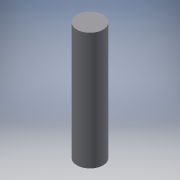
# Autodesk Inventor part: cil_sierra
Saved by Autodesk Inventor 2018 (Build 220112000, 112)
## iProperties
Created: 2021-07-10
Part Number: cil_sierra
Material: Genérico
Document SubType Name: Modeling
Designer: GABRIEL
Density: 1 g/cm^3
Appearance: Valor por defecto
Author: GABRIEL
Autodesk Inventor part; units mm, degrees
ref_plane "YZ Plane" through (0, 0, 0) normal (1, 0, 0) x (0, 1, 0)
ref_plane "XZ Plane" through (0, 0, 0) normal (0, 1, 0) x (-1, 0, 0)
ref_plane "XY Plane" through (0, 0, 0) normal (0, 0, 1) x (1, 0, 0)
sketch "Boceto1" plane through (0, 0, 0) normal (0, 0, 1) x (1, 0, 0)
  circle A0 centre (0, 0) radius 10
  dimension "d0" = 20
  constraints: 1 centre point, 1 coincident
  measures "d0" diameter of A0
extrude "Extrusión1" add sketch "Boceto1" along normal blind 110
sketch "Boceto2" plane through (0, 0, 110) normal (0, 0, 1) x (1, 0, 0)
  line L0 (2.5, -6) -> (-2.5, -6)
  line L1 (-2.5, -6) -> (-2.5, 6)
  line L2 (-2.5, 6) -> (2.5, 6)
  line L3 (2.5, 6) -> (2.5, -6)
  line L4 (2.5, -6) -> (-2.5, 6) construction
  line L5 (-2.5, -6) -> (2.5, 6) construction
  point P0 (0, 0)
  dimension "d3" = 5
  dimension "d4" = 12
  constraints: 12 end point, 2 midpoint, 2 parallel, 1 horizontal, 1 perpendicular
  measures "d3" distance of L1.end L2.end
  measures "d4" distance of L0.end L1.end
extrude "Extrusión2" add sketch "Boceto2" along normal blind 30
sketch "Boceto3" plane through (-2.5, -6, 110) normal (-1, 0, 0) x (0, 0, 1)
  circle A0 centre (24, 6) radius 4
  line L0 (30, 12) -> (30, 0) projected
  line L1 (0, 12) -> (30, 12) projected
  point P0 (-110, 6)
  dimension "d7" = 8
  dimension "d8" = 6
  dimension "d9" = 6
  constraints: 1 centre point
  measures "d7" diameter of A0
  measures "d8" distance from line of L0 A0.centre
  measures "d9" distance from line of L1 A0.centre
extrude "Extrusión3" cut sketch "Boceto3" against normal blind 30
